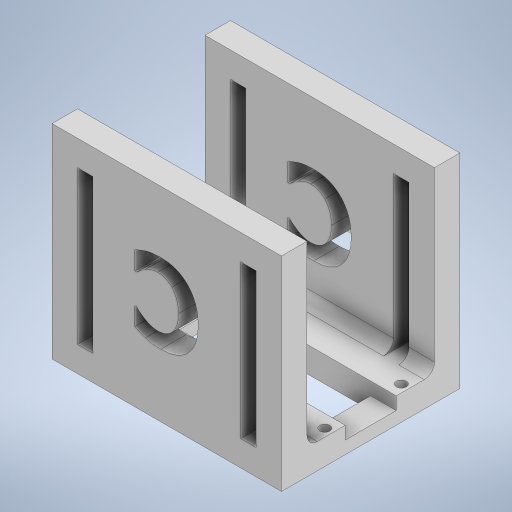
# Autodesk Inventor part: nano
Saved by Autodesk Inventor 2024 (Build 280153000, 153)
## iProperties
Created: 2024-03-29
Part Number: nano
Material: Generic
Document SubType Name: Modeling
Designer: JDAM
Mass: 19.017 g
Surface Area: 107.933 cm^2
Volume: 19.017 cm^3
Density: 1 g/cm^3
Appearance: Default
Author: JDAM
Autodesk Inventor part; units mm, degrees
ref_plane "YZ Plane" through (0, 0, 0) normal (1, 0, 0) x (0, 1, 0)
ref_plane "XZ Plane" through (0, 0, 0) normal (0, 1, 0) x (-1, 0, 0)
ref_plane "XY Plane" through (0, 0, 0) normal (0, 0, 1) x (1, 0, 0)
sketch "Sketch1" plane through (0, 0, 0) normal (0, 1, 0) x (-1, 0, 0)
  line L0 (22.5, 12.5) -> (-22.5, 12.5)
  line L1 (-22.5, 12.5) -> (-22.5, -12.5)
  line L2 (-22.5, -12.5) -> (22.5, -12.5)
  line L3 (22.5, -12.5) -> (22.5, 12.5)
  line L4 (22.5, 12.5) -> (-22.5, -12.5) construction
  line L5 (-22.5, 12.5) -> (22.5, -12.5) construction
  line L6 (-17.5, 5) -> (17.5, 5)
  line L7 (17.5, 5) -> (17.5, -5)
  line L8 (17.5, -5) -> (-17.5, -5)
  line L9 (-17.5, -5) -> (-17.5, 5)
  line L10 (-17.5, 5) -> (17.5, -5) construction
  line L11 (17.5, 5) -> (-17.5, -5) construction
  line L12 (-17.5, 5) -> (-22.5, 5)
  line L13 (-17.5, -5) -> (-22.5, -5)
  line L14 (12.5, 0) -> (12.5, -5)
  line L15 (12.5, 0) -> (12.5, 5)
  point P0 (0, 0)
  dimension "d0" = 45
  dimension "d1" = 25
  dimension "d4" = 35
  dimension "d5" = 10
  constraints: 32 end point, 5 perpendicular, 5 point on line, 4 midpoint, 4 parallel, 2 horizontal
  measures "d0" distance of L2.end L1.end
  measures "d1" distance of L1.end L0.end
  measures "d4" distance of L7.end L8.end
  measures "d5" distance of L6.end L7.end
extrude "Extrusion1" add sketch "Sketch1" along normal blind 5 contours L3 L2 L1 L13 L8 L7 L6 L12 L0
extrude "Extrusion2" add sketch "Sketch1" along normal blind 2.5 contours L12 L9 L13 L1
extrude "Extrusion3" add sketch "Sketch1" along normal blind 2.5 contours L6 L7 L8 L14 L15
sketch "Sketch2" plane through (0, 0, 0) normal (0, 1, 0) x (-1, 0, 0)
  line L0 (-22.5, -12.5) -> (22.5, -12.5) projected
  line L1 (22.5, -12.5) -> (-22.5, -12.5)
  line L2 (-22.5, -12.5) -> (-22.5, -17.5)
  line L3 (-22.5, -17.5) -> (22.5, -17.5)
  line L4 (22.5, -17.5) -> (22.5, -12.5)
  point P0 (0, 0)
  point P1 (-22.5, -12.5)
  dimension "d13" = 45
  dimension "d14" = 5
  constraints: 8 end point, 2 parallel, 1 horizontal, 1 perpendicular
  measures "d13" distance of L3.end L2.end
  measures "d14" distance of L2.end L1.end
extrude "Extrusion4" add sketch "Sketch2" along normal blind 40
mirror "Mirror1" about plane through (0, 0, 0) normal (0, 0, 1) of "Extrusion4"
sketch "Sketch3" plane through (22.5, 0, -17.5) normal (0, 0, -1) x (-1, 0, 0)
  line L0 (0, 0) -> (0, 40) projected
  line L1 (0, 40) -> (5, 40)
  line L2 (0, 40) -> (45, 40) projected
  line L3 (5, 40) -> (5, 35)
  line L4 (0, 20) -> (45, 20)
  line L5 (45, 0) -> (45, 40) projected
  line L6 (0, 0) -> (5, 0)
  line L7 (5, 0) -> (5, 5)
  line L8 (0, 5) -> (45, 5) projected
  line L9 (5, 35) -> (8, 35)
  line L10 (8, 35) -> (8, 5)
  line L11 (8, 5) -> (5, 5)
  line L12 (5, 5) -> (5, 35)
  line L13 (22.5, 0) -> (22.5, 40)
  line L14 (40, 35) -> (37, 35)
  line L15 (37, 35) -> (37, 5)
  line L16 (37, 5) -> (40, 5)
  line L17 (40, 5) -> (40, 35)
  dimension "d17" = 5
  dimension "d18" = 5
  dimension "d19" = 3
  constraints: 28 end point, 6 symmetric about line, 3 midpoint, 2 parallel, 2 point on line, 1 horizontal, 1 perpendicular, 1 vertical
  measures "d17" distance of L0.end L1.end
  measures "d18" distance of L1.end L3.end
  measures "d19" distance of L10.end L11.end
extrude "Extrusion5" cut sketch "Sketch3" against normal blind 40 contours L12 L4 L10 L8 | L12 L9 L10 L4 | L15 L4 L17 L8 | L15 L14 L17 L4
fillet "Fillet1" radius 2 6 edges at (20, 5, 12.5) (0, 5, 12.5) (-20, 5, 12.5) (20, 5, -12.5) (0, 5, -12.5) (-20, 5, -12.5)
ref_plane "Work Plane1" through (-0.618, 26.6153, -17.5) normal (0, 0, -1) x (-1, 0, 0)
sketch "Sketch11" plane through (0, 5, 0) normal (0, 1, 0) x (1, 0, 0)
  line L0 (-17.4182, 0) -> (-19.9182, 0)
  line L1 (22, -8.5) -> (-22, -8.5)
  line L2 (-22, -8.5) -> (-22, 8.5)
  line L3 (-22, 8.5) -> (22, 8.5)
  line L4 (22, 8.5) -> (22, -8.5)
  line L5 (22, -8.5) -> (-22, 8.5) construction
  line L6 (-22, -8.5) -> (22, 8.5) construction
  line L7 (-22, 8.5) -> (-22, 6.5)
  line L8 (-22, 7.5) -> (-20, 7.5)
  circle A0 centre (-21, 7.5) radius 1
  point P0 (0, 0)
  dimension "d35" = 2.5
  dimension "d36" = 44
  dimension "d37" = 17
  dimension "d38" = 2
  dimension "d39" = 2
  dimension "d40" = 2
  constraints: 18 end point, 4 midpoint, 3 horizontal, 2 parallel, 1 centre point, 1 perpendicular, 1 point on line
  measures "d35" distance of L0.start L0.end
  measures "d36" distance of L2.end L3.end
  measures "d37" distance of L1.end L2.end
  measures "d38" distance of L2.end L7.end
  measures "d39" distance of L8.start L8.end
  measures "d40" diameter of A0
hole "Hole1" at (-21, 5, -7.5) direction (0, -1, 0) diameter 2 depth 12.7625
mirror "Mirror2" about plane through (0, 0, 0) normal (0, 0, 1) of "Hole1"
mirror "Mirror3" about plane through (0, 0, 0) normal (1, 0, 0) of "Hole1", "Mirror2"
sketch "Sketch12" plane through (22.5, 0, -17.5) normal (0, 0, -1) x (-1, 0, 0)
  line L0 (8.0654, 34.9544) -> (36.9904, 34.9544) construction
  line L1 (36.9904, 34.9544) -> (36.9904, 5.3063) construction
  line L2 (36.9904, 5.3063) -> (8.0654, 5.3063) construction
  line L3 (8.0654, 5.3063) -> (8.0654, 34.9544) construction
  spline S0 degree 2 poles (23.6644, 12.3386) (20.2852, 12.3386) (16.3225, 16.4229) (16.3225, 20.1182) knots 0 0 0 1 2 2 2
  spline S1 degree 2 poles (16.3225, 20.1182) (16.3225, 23.6798) (20.2973, 27.9221) (23.6766, 27.9221) knots 0 0 0 1 2 2 2
  spline S2 degree 2 poles (23.6766, 27.9221) (24.564, 27.9221) (25.9983, 27.7154) (26.6547, 27.5453) knots 0 0 0 1 2 2 2
  spline S3 degree 2 poles (26.6547, 27.5453) (27.1652, 27.3872) (28.3687, 26.8645) (28.7455, 26.6701) knots 0 0 0 1 2 2 2
  line L4 (28.7455, 26.6701) -> (28.7455, 23.0963)
  line L5 (28.7455, 23.0963) -> (28.3687, 23.0963)
  spline S4 degree 2 poles (28.3687, 23.0963) (28.0891, 23.3394) (27.2625, 24.0201) (26.7398, 24.3362) knots 0 0 0 1 2 2 2
  spline S5 degree 2 poles (26.7398, 24.3362) (26.2171, 24.6644) (24.9651, 25.1141) (24.2722, 25.1141) knots 0 0 0 1 2 2 2
  spline S6 degree 2 poles (24.2722, 25.1141) (23.4578, 25.1141) (22.1085, 24.6036) (21.4886, 23.9594) knots 0 0 0 1 2 2 2
  spline S7 degree 2 poles (21.4886, 23.9594) (20.9294, 23.388) (20.2122, 21.431) (20.2122, 20.106) knots 0 0 0 1 2 2 2
  spline S8 degree 2 poles (20.2122, 20.106) (20.2122, 18.7081) (20.9537, 16.7997) (21.5615, 16.2162) knots 0 0 0 1 2 2 2
  spline S9 degree 2 poles (21.5615, 16.2162) (22.145, 15.6449) (23.5793, 15.1466) (24.2965, 15.1466) knots 0 0 0 1 2 2 2
  spline S10 degree 2 poles (24.2965, 15.1466) (25.038, 15.1466) (26.3873, 15.6449) (26.8492, 15.9488) knots 0 0 0 1 2 2 2
  spline S11 degree 2 poles (26.8492, 15.9488) (27.3597, 16.2527) (28.1255, 16.897) (28.4051, 17.1522) knots 0 0 0 1 2 2 2
  line L6 (28.4051, 17.1522) -> (28.7455, 17.1522)
  line L7 (28.7455, 17.1522) -> (28.7455, 13.6271)
  spline S12 degree 2 poles (28.7455, 13.6271) (28.3322, 13.4326) (27.2503, 12.9464) (26.6669, 12.7762) knots 0 0 0 1 2 2 2
  spline S13 degree 2 poles (26.6669, 12.7762) (25.9618, 12.5574) (24.7341, 12.3386) (23.6644, 12.3386) knots 0 0 0 1 2 2 2
  point P0 (22.5, 0)
  constraints: 2 other
extrude "Extrusion11" cut sketch "Sketch12" against normal blind 40
body "Solid1"
